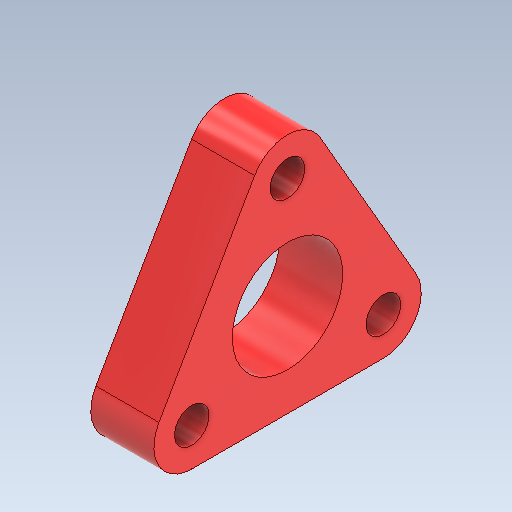
# Autodesk Inventor part: Part2
Saved by Autodesk Inventor 2021 (Build 250183000, 183)
## iProperties
Created: 2022-04-30
Part Number: Part2
Material: Generic
Document SubType Name: Modeling
Designer: authe
Density: 1 g/cm^3
Appearance: Light Red
Author: authe
Autodesk Inventor part; units mm, degrees
ref_plane "YZ Plane" through (0, 0, 0) normal (1, 0, 0) x (0, 1, 0)
ref_plane "XZ Plane" through (0, 0, 0) normal (0, 1, 0) x (-1, 0, 0)
ref_plane "XY Plane" through (0, 0, 0) normal (0, 0, 1) x (1, 0, 0)
sketch "Sketch1" plane through (0, 0, 0) normal (1, 0, 0) x (0, 1, 0)
  point P0 (0, 0)
sketch "Sketch2" plane through (0, 0, 0) normal (1, 0, 0) x (0, 1, 0)
  circle A0 centre (0, 0) radius 17.5
  circle A1 centre (35.0665, 0.0228) radius 5.5
  circle A2 centre (-17.553, 30.3571) radius 5.5
  circle A3 centre (-17.5135, -30.3799) radius 5.5
  circle A4 centre (-17.5135, -30.3799) radius 12
  circle A5 centre (35.0665, 0.0228) radius 12
  circle A6 centre (-17.553, 30.3571) radius 12
  line L0 (-29.5135, -30.3877) -> (-29.553, 30.3493)
  line L1 (-11.5597, 40.7533) -> (41.0597, 10.419)
  line L2 (41.0732, -10.3656) -> (-11.5068, -40.7683)
  arc A7 (34.6387, -5.4605) -> (34.6316, 5.5056) centre (0, 0) ccw
  arc A8 (-26.717, 22.6098) -> (-29.5455, 18.7634) centre (0, 0) ccw
  arc A9 (-29.521, -18.8018) -> (-26.6876, -22.6445) centre (0, 0) ccw
  arc A10 (31.0434, -16.1651) -> (32.9545, -11.7899) centre (0, 0) ccw
  dimension "d0" = 35
  dimension "d2" = 11
  dimension "d5" = 360
  dimension "d7" = 24
  dimension "d8" = 24
  dimension "d9" = 24
  constraints: 20 point on circle, 11 centre point, 6 coincident, 6 end point, 3 point on line, 2 tangent, 11 other
  measures "d0" diameter of A0
  measures "d2" diameter of A1
  measures "d7" diameter of A4
  measures "d8" diameter of A5
  measures "d9" diameter of A6
extrude "Extrusion1" add sketch "Sketch2" along normal blind 20
body "Solid1"
